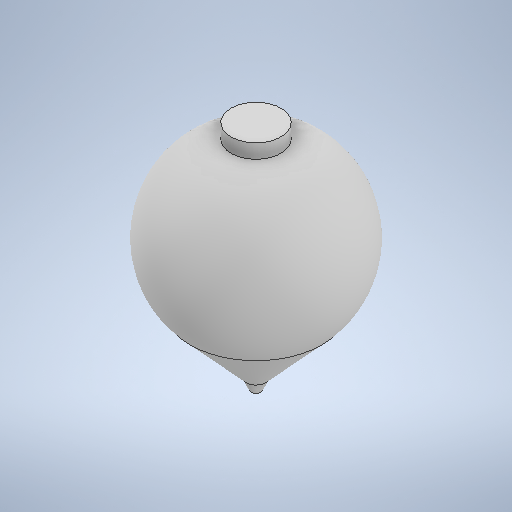
# Autodesk Inventor part: Peça6
Saved by Autodesk Inventor 2025.2 (Build 292293000, 293)
## iProperties
Created: 2025-03-25
Part Number: Peça6
Material: Genérico
Document SubType Name: Modeling
Designer: Formação
Density: 1 g/cm^3
Appearance: Padrão
Author: Formação
Autodesk Inventor part; units mm, degrees
ref_plane "YZ Plane" through (0, 0, 0) normal (1, 0, 0) x (0, 1, 0)
ref_plane "XZ Plane" through (0, 0, 0) normal (0, 1, 0) x (-1, 0, 0)
ref_plane "XY Plane" through (0, 0, 0) normal (0, 0, 1) x (1, 0, 0)
sketch "Esboço1" plane through (0, 0, 0) normal (0, 0, 1) x (1, 0, 0)
  circle A0 centre (0, 0) radius 12.5 construction
  line L0 (9.1994, -8.4629) -> (0, -18.4629) construction
  line L1 (-3.5, 14) -> (3.5, 13.9971) construction
  line L2 (-3.5, 14) -> (-3.5, 12) construction
  line L3 (0, 13.9985) -> (-3.5, 14)
  line L4 (-3.5, 14) -> (-3.5, 12)
  arc A1 (-3.5, 12) -> (-9.1994, -8.4629) centre (0, 0) ccw
  line L5 (0, 13.9985) -> (0, -18.4629)
  line L6 (-3.5, 13.5) -> (0, 13.5)
  line L7 (-3.5, 13) -> (0, 13)
  line L8 (-1.3799, -16.9629) -> (0, -16.9629) construction
  line L9 (-1.3799, -16.9629) -> (-1.3799, -18.4629) construction
  line L10 (-9.1994, -8.4629) -> (-1.3799, -16.9629)
  line L11 (-1.3799, -16.9629) -> (-1.3799, -18.4629) construction
  line L12 (0, -18.4629) -> (-1.3799, -18.4629) construction
  line L13 (-1.3799, -16.9629) -> (-0.69, -18.4629)
  line L14 (-0.69, -18.4629) -> (0, -18.4629)
  line L15 (0, -24.9555) -> (0, 20.4926) projected
  point P0 (-1.75, 13.5)
  point P1 (-1.75, 13)
  dimension "d0" = 25
  dimension "d4" = 7
  dimension "d5" = 2
  dimension "d6" = 32.46
  dimension "d9" = 10
  dimension "d10" = 0.5
  dimension "d11" = 1.5
  constraints: 30 end point, 5 midpoint, 5 perpendicular, 5 point on circle, 4 point on line, 3 coincident, 3 collinear, 3 vertical, 3 vertical alignment, 2 centre point, 2 tangent, 1 horizontal alignment
  measures "d0" diameter of A0
  measures "d4" distance of L1.end L1.start
  measures "d5" distance of L2.end L1.start
  measures "d6" vertical distance of L0.end L1.end
  measures "d9" vertical distance of L0.end L10.start
  measures "d10" distance between parallel lines of L7 L6
  measures "d11" distance of L9.end L8.start
revolve "Revolução1" add sketch "Esboço1" angle 360 about axis through (0, -10, 0) along (0, 1, 0)
